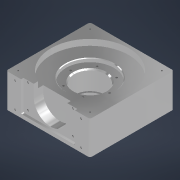
# Autodesk Inventor part: Soporte
Saved by Autodesk Inventor 2022 (Build 260153000, 153)
## iProperties
Created: 2021-09-20
Part Number: Soporte
Material: Aluminum 6061
Document SubType Name: Modeling
Designer: Andres
Density: 2.7 g/cm^3
Appearance: Aluminum - Flat
Author: Andres
Autodesk Inventor part; units mm, degrees
ref_plane "YZ Plane" through (0, 0, 0) normal (1, 0, 0) x (0, 1, 0)
ref_plane "XZ Plane" through (0, 0, 0) normal (0, 1, 0) x (-1, 0, 0)
ref_plane "XY Plane" through (0, 0, 0) normal (0, 0, 1) x (1, 0, 0)
sketch "Sketch1" plane through (0, 0, 0) normal (0, 1, 0) x (-1, 0, 0)
  circle A0 centre (0, 0) radius 65
  line L0 (-70, 70) -> (70, 70)
  line L1 (70, 70) -> (70, -70)
  line L2 (70, -70) -> (-70, -70)
  line L3 (-70, -70) -> (-70, 70)
  line L4 (-70, 70) -> (70, -70) construction
  line L5 (70, 70) -> (-70, -70) construction
  circle A1 centre (0, 0) radius 23
  dimension "d0" = 130
  dimension "d1" = 140
  dimension "d2" = 140
  dimension "Db" = 46
  constraints: 12 end point, 2 centre point, 2 coincident, 2 midpoint, 2 parallel, 1 horizontal, 1 perpendicular
  measures "d0" diameter of A0
  measures "d1" distance of L1.end L2.end
  measures "d2" distance of L0.end L1.end
  measures "Db" diameter of A1
extrude "Extrusion1" add sketch "Sketch1" along normal blind 10 contours L0 L1 L2 L3
extrude "Extrusion2" add sketch "Sketch1" against normal blind 46 contours A0 | L0 L1 L2 L3
sketch "Sketch2" plane through (0, 0, 0) normal (0, 1, 0) x (1, 0, 0)
  circle A0 centre (0, 0) radius 26
  circle A1 centre (0, 0) radius 23 projected
  dimension "d8" = 52
  constraints: 1 centre point, 1 coincident
  measures "d8" diameter of A0
extrude "Extrusion3" cut sketch "Sketch2" against normal blind 38
sketch "Plate Mounting Holes" plane through (-70, 10, 70) normal (0, 0, 1) x (1, 0, 0)
  line L0 (140, -56) -> (140, 0) construction
  line L1 (0, 0) -> (140, 0) construction
  line L2 (0, -56) -> (0, 0) construction
  line L3 (140, -56) -> (0, -56) construction
  line L4 (30, -51) -> (110, -51) construction
  line L5 (110, -51) -> (110, -5) construction
  line L6 (110, -5) -> (30, -5) construction
  line L7 (30, -5) -> (30, -51) construction
  line L8 (30, -51) -> (110, -5) construction
  line L9 (110, -51) -> (30, -5) construction
  point P0 (70, -10)
  point P1 (70, -28)
  point P2 (70, -28)
  point P3 (70, 0)
  dimension "d14" = 5
  dimension "d15" = 5
  dimension "d16" = 80
  constraints: 12 end point, 4 coincident, 4 midpoint, 2 parallel, 1 horizontal, 1 perpendicular, 1 vertical alignment
  measures "d14" distance between parallel lines of L1 L6
  measures "d15" distance between parallel lines of L3 L4
  measures "d16" distance between parallel lines of L5 L7
sketch "PlateHole" plane through (-70, 10, 70) normal (0, 0, 1) x (1, 0, 0)
  line L0 (42, -51) -> (98, -51)
  line L1 (98, -51) -> (98, 0)
  line L2 (98, 0) -> (42, 0)
  line L3 (42, 0) -> (42, -51)
  line L4 (42, -51) -> (98, 0) construction
  line L5 (98, -51) -> (42, 0) construction
  line L6 (140, -56) -> (0, -56) projected
  line L7 (0, 0) -> (140, 0) projected
  circle A0 centre (70, -20) radius 28
  point P0 (70, -10)
  point P1 (70, -25.5)
  point P2 (70, -28)
  point P3 (70, -25.5)
  point P4 (42, -20)
  point P5 (98, -20)
  dimension "d18" = 5
  dimension "d24" = 20
  dimension "d25" = 56
  constraints: 12 end point, 3 midpoint, 2 parallel, 2 tangent, 1 centre point, 1 collinear, 1 horizontal, 1 perpendicular, 1 vertical alignment
  measures "d18" distance between parallel lines of L6 L0
  measures "d24" distance from line of L7 A0.centre
  measures "d25" distance between parallel lines of L1 L3
sketch "Sketch7" plane through (0, 0, 0) normal (0, 1, 0) x (1, 0, 0)
  circle A0 centre (0, 0) radius 26 projected
  circle A1 centre (0, 0) radius 26 projected
  circle A2 centre (0, 0) radius 40
  dimension "d19" = 80
  constraints: 1 centre point, 1 coincident
  measures "d19" diameter of A2
extrude "Extrusion4" cut sketch "Sketch7" against normal blind 6
extrude "Extrusion5" cut sketch "PlateHole" against normal blind 20 contours L3 L2 A0 | A0 L2 | A0 L2 L1 picked at (77.8067, -22.9554)
chamfer "Chamfer2" distance 2 angle 45 1 edges at (-26, -6, 0)
chamfer "Chamfer3" distance 1 angle 45 1 edges at (-40, 0, 0)
sketch "Sketch10" plane through (0, -6, 0) normal (0, 1, 0) x (1, 0, 0)
  circle A0 centre (16.25, 28.1458) radius 3.25 projected
  circle A1 centre (16.25, -28.1458) radius 3.25 projected
  circle A2 centre (-32.5, 0) radius 3.25 projected
  circle A3 centre (-16.25, -28.1458) radius 3.25 projected
  circle A4 centre (32.5, 0) radius 3.25 projected
  circle A5 centre (-16.25, 28.1458) radius 3.25 projected
  circle A6 centre (0, 0) radius 39 projected
  circle A7 centre (0, 0) radius 24.5 projected
hole "Hole2" at (-32.5, -6, 0) at (-16.25, -6, 28.1458) at (16.25, -6, 28.1458) at (32.5, -6, 0) at (16.25, -6, -28.1458) at (-16.25, -6, -28.1458) direction (0, -1, 0) diameter 3.242 depth 11.8 tip angle 118 thread size "M4x0.7" class "6H" standard "ISO Metric profile"
sketch "Sketch11" plane through (-70, -46, 70) normal (0, 0, 1) x (1, 0, 0)
  line L0 (98, 56) -> (98, 36) projected
  arc A0 (42, 36) -> (98, 36) centre (70, 36) ccw projected
  line L1 (42, 36) -> (42, 56) projected
  line L2 (0, 56) -> (42, 56) projected
  line L3 (0, 0) -> (0, 56) projected
  line L4 (140, 0) -> (0, 0) projected
  line L5 (140, 0) -> (140, 56) projected
  line L6 (98, 56) -> (140, 56) projected
  arc A1 (42, 36) -> (98, 36) centre (70, 36) ccw projected
  line L7 (25, 6) -> (115, 6)
  line L8 (25, 6) -> (25, 56)
  line L9 (115, 6) -> (115, 56)
  line L10 (140, 56) -> (0, 56) projected
  point P0 (70, 46)
  point P1 (70, 6)
  point P2 (115, 56)
  dimension "d50" = 30
  dimension "d51" = 90
  constraints: 6 end point, 2 perpendicular, 2 point on line, 1 horizontal, 1 midpoint, 1 vertical, 1 vertical alignment
  measures "d50" distance from line of L7 A0.centre
  measures "d51" distance between parallel lines of L9 L8
extrude "Extrusion6" cut sketch "Sketch11" against normal blind 4 contours L6 L9 L7 L8 L2 L1 A0 L0
fillet "Fillet1" radius 2 2 edges at (45, -40, 68) (-45, -40, 68)
sketch "Sketch13" plane through (-70, -46, 66) normal (0, 0, 1) x (1, 0, 0)
  circle A0 centre (32.5, 53) radius 2.25 projected
  circle A1 centre (32.5, 13) radius 2.25 projected
  circle A2 centre (107.5, 13) radius 2.25 projected
  circle A3 centre (107.5, 53) radius 2.25 projected
  point P0 (70, 46)
hole "Hole3" at (-37.5, 7, 66) at (-37.5, -33, 66) at (37.5, -33, 66) at (37.5, 7, 66) direction (0, 0, -1) diameter 3.242 depth 10 tip angle 118 thread size "M4x0.7" class "6H" standard "ISO Metric profile"
chamfer "Chamfer5" distance 4 angle 45 1 edges at (23, -46, 0)
sketch "Sketch14" plane through (0, 10, 0) normal (0, 1, 0) x (1, 0, 0)
  circle A0 centre (60, 60) radius 3.25 projected
  circle A1 centre (-60, -60) radius 3.25 projected
  circle A2 centre (-60, 60) radius 3.25 projected
  circle A3 centre (60, -60) radius 3.25 projected
  line L0 (45, -66) -> (45, -70) projected
  line L1 (45, -70) -> (67, -70) projected
  line L2 (70, -67) -> (70, 67) projected
  line L3 (67, 70) -> (-67, 70) projected
  line L4 (-70, 67) -> (-70, -67) projected
  line L5 (-67, -70) -> (-45, -70) projected
  line L6 (-45, -70) -> (-45, -66) projected
  line L7 (-45, -66) -> (45, -66) projected
  circle A4 centre (0, 0) radius 24.5 projected
  arc A5 (67, -70) -> (70, -67) centre (67, -67) ccw projected
  arc A6 (70, 67) -> (67, 70) centre (67, 67) ccw projected
  arc A7 (-67, 70) -> (-70, 67) centre (-67, 67) ccw projected
  arc A8 (-70, -67) -> (-67, -70) centre (-67, -67) ccw projected
  point P0 (0, 0)
hole "Hole4" at (-60, 10, 60) at (60, 10, 60) at (60, 10, -60) at (-60, 10, -60) direction (0, -1, 0) diameter 2.459 depth 8.8 tip angle 118 thread size "M3x0.5" class "6H" standard "ISO Metric profile"
fillet "Fillet2" radius 3 4 edges at (70, -18, 70) (70, -18, -70) (-70, -18, -70) (-70, -18, 70)
sketch "Sketch15" plane through (67, 10, -70) normal (0, 0, -1) x (-1, 0, 0)
  line L0 (12, -49) -> (122, -49) construction
  line L1 (122, -49) -> (122, -7) construction
  line L2 (122, -7) -> (12, -7) construction
  line L3 (12, -7) -> (12, -49) construction
  line L4 (12, -49) -> (122, -7) construction
  line L5 (122, -49) -> (12, -7) construction
  line L6 (0, -56) -> (0, 0) construction
  point P0 (67, -10)
  point P1 (67, -28)
  point P2 (0, -28)
  dimension "d73" = 110
  dimension "d74" = 42
  constraints: 12 end point, 3 midpoint, 2 parallel, 1 horizontal, 1 horizontal alignment, 1 perpendicular, 1 vertical alignment
  measures "d73" distance between parallel lines of L1 L3
  measures "d74" distance between parallel lines of L0 L2
hole "Hole5" at (55, 3, -70) at (55, -39, -70) at (-55, -39, -70) at (-55, 3, -70) direction (0, 0, 1) diameter 3.242 depth 11.8 tip angle 118 thread size "M4x0.7" class "6H" standard "ISO Metric profile"
sketch "Sketch16" plane through (-43, -40, 70) normal (0, 0, 1) x (1, 0, 0)
  circle A0 centre (-12, 1) radius 1.621 projected
  circle A1 centre (98, 43) radius 1.621 projected
  circle A2 centre (98, 1) radius 1.621 projected
  circle A3 centre (-12, 43) radius 1.621 projected
  line L0 (-24, 50) -> (-24, -6) projected
  line L1 (110, 50) -> (-24, 50) projected
  line L2 (110, -6) -> (110, 50) projected
  line L3 (-24, -6) -> (110, -6) projected
  point P0 (43, 40)
hole "Hole6" at (-55, 3, 70) at (-55, -39, 70) at (55, -39, 70) at (55, 3, 70) direction (0, 0, -1) diameter 3.242 depth 11.8 tip angle 118 thread size "M4x0.7" class "6H" standard "ISO Metric profile"
equation "\"d15\" = d14"
body "Solid1"
